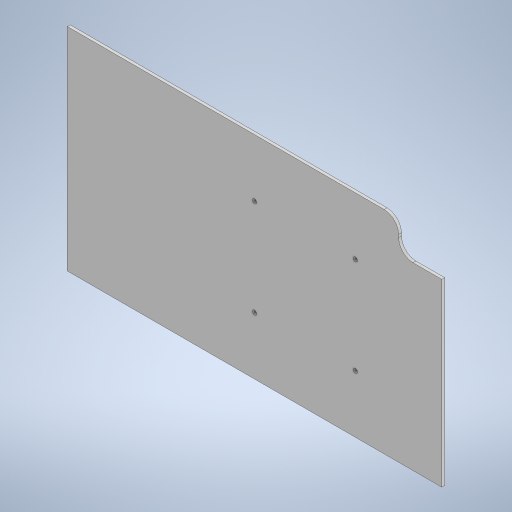
# Autodesk Inventor part: Coffee_Machine_Base
Saved by Autodesk Inventor 2023.5 (Build 275446020, 446B)
## iProperties
Created: 2025-04-17
Part Number: Coffee_Machine_Base
Material: Generic
Document SubType Name: Modeling
Designer: Lucky Sah
Density: 1 g/cm^3
Appearance: Default
Author: Lucky Sah
Autodesk Inventor part; units mm, degrees
ref_plane "YZ Plane" through (0, 0, 0) normal (1, 0, 0) x (0, 1, 0)
ref_plane "XZ Plane" through (0, 0, 0) normal (0, 1, 0) x (-1, 0, 0)
ref_plane "XY Plane" through (0, 0, 0) normal (0, 0, 1) x (1, 0, 0)
sketch "Sketch1" plane through (0, 0, 0) normal (0, 0, 1) x (1, 0, 0)
  line L0 (0, 0) -> (260, 0)
  line L1 (260, 0) -> (260, 125)
  line L2 (220, 147) -> (0, 147)
  line L3 (0, 147) -> (0, 0)
  circle A0 centre (240, 135) radius 8
  circle A1 centre (240, 135) radius 10
  line L4 (250, 135) -> (250.202, 135)
  line L5 (230, 135) -> (230, 137)
  arc A2 (230, 137) -> (220, 147) centre (220, 137) ccw
  line L6 (260, 147) -> (260, 147)
  line L7 (250, 135) -> (250, 137)
  line L8 (240, 125) -> (260, 125)
  line L9 (0, 73.5) -> (260, 73.5)
  line L10 (60, 107) -> (200, 107)
  line L11 (200, 107) -> (200, 40)
  line L12 (200, 40) -> (60, 40)
  line L13 (60, 40) -> (60, 107)
  circle A3 centre (60, 107) radius 1.5
  circle A4 centre (200, 107) radius 1.5
  circle A5 centre (200, 40) radius 1.5
  circle A6 centre (60, 40) radius 1.5
  circle A7 centre (130, 107) radius 1.5
  circle A8 centre (130, 40) radius 1.5
  line L14 (260, 125) -> (264, 125)
  line L15 (264, 125) -> (264, 0)
  line L16 (264, 0) -> (260, 0)
  line L17 (260, 0) -> (260, 125)
  line L18 (0, 147) -> (-4, 147)
  line L19 (-4, 147) -> (-4, 0)
  line L20 (-4, 0) -> (0, 0)
  line L21 (0, 0) -> (0, 147)
  line L22 (-4, 147) -> (-44, 147)
  line L23 (-54, 137) -> (-54, 10)
  line L24 (-44, 0) -> (-4, 0)
  line L25 (-4, 0) -> (-4, 147)
  line L26 (264, 125) -> (304, 125)
  line L27 (314, 115) -> (314, 10)
  line L28 (304, 0) -> (264, 0)
  line L29 (264, 0) -> (264, 125)
  arc A9 (-44, 147) -> (-54, 137) centre (-44, 137) ccw
  arc A10 (-54, 10) -> (-44, 0) centre (-44, 10) ccw
  arc A11 (304, 0) -> (314, 10) centre (304, 10) ccw
  arc A12 (314, 115) -> (304, 125) centre (304, 115) ccw
  point P0 (260, 67.5)
  point P1 (-54, 0)
  point P2 (314, 0)
  dimension "d2" = 16
  dimension "d3" = 20
  dimension "d4" = 135
  dimension "d5" = 2
  dimension "d6" = 260
  dimension "d7" = 147
  dimension "d8" = 10
  dimension "d11" = 22
  dimension "d16" = 40
  dimension "d17" = 40
  dimension "d18" = 60
  dimension "d19" = 60
  dimension "d20" = 3
  dimension "d21" = 3
  dimension "d22" = 3
  dimension "d23" = 3
  dimension "d24" = 140
  dimension "d25" = 67
  dimension "d26" = 3
  dimension "d27" = 3
  dimension "d29" = 70
  dimension "d30" = 4
  dimension "d31" = 4
  dimension "d32" = 50
  dimension "d33" = 50
  dimension "d34" = 10
  dimension "d35" = 368
  constraints: 62 end point, 13 centre point, 13 point on circle, 12 parallel, 12 tangent, 11 perpendicular, 10 point on line, 6 horizontal, 4 coincident, 3 equal radius, 3 midpoint, 1 collinear
  measures "d2" diameter of A0
  measures "d3" distance from line of L1 A0.centre
  measures "d4" distance from line of L0 A0.centre
  measures "d5" radial gap between concentric circles of A0 A1
  measures "d6" distance from line of point (260, 67.5) L3
  measures "d7" distance between parallel lines of L0 L2
  measures "d8" radius of A2
  measures "d11" distance between parallel lines of L2 L8
  measures "d16" distance between parallel lines of L10 L2
  measures "d17" distance between parallel lines of L0 L12
  measures "d18" distance between parallel lines of L3 L13
  measures "d19" distance between parallel lines of L1 L11
  measures "d20" diameter of A3
  measures "d21" diameter of A4
  measures "d22" diameter of A5
  measures "d23" diameter of A6
  measures "d24" distance between parallel lines of L11 L13
  measures "d25" distance between parallel lines of L12 L10
  measures "d26" diameter of A7
  measures "d27" diameter of A8
  measures "d29" distance from line of L11 A8.centre
  measures "d30" distance between parallel lines of L15 L1
  measures "d31" distance between parallel lines of L19 L3
  measures "d32" distance between parallel lines of L23 L19
  measures "d33" distance between parallel lines of L27 L15
  measures "d34" radius of A9
  measures "d35" distance between parallel lines of L27 L23
extrude "Extrusion1" add sketch "Sketch1" along normal blind 2 contours L3 L9 L13 A6 L12 A8 A5 L11 L1 L0 | L3 L2 A2 L5 A1 L8 L1 L9 L11 A4 L10 A7 A3 L13 | L13 A3 L10 A7 A4 L11 L9 | L9 L11 A5 L12 A8 A6 L13 | A6 L12 L13 | L13 L12 A6 | A3 L10 L13 | L13 L10 A3
body "Solid1"
